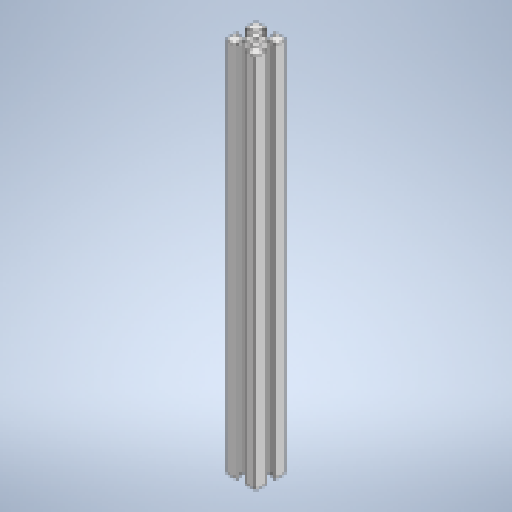
# Autodesk Inventor part: j2j3 alumi ext
Saved by Autodesk Inventor 2025 (Build 290162000, 162)
## iProperties
Created: 2025-07-28
Part Number: j2j3 alumi ext
Material: 一般
Document SubType Name: Modeling
Designer: gavin
Density: 1 g/cm^3
Appearance: 預設
Author: gavin
Autodesk Inventor part; units mm, degrees
ref_plane "YZ Plane" through (0, 0, 0) normal (1, 0, 0) x (0, 1, 0)
ref_plane "XZ Plane" through (0, 0, 0) normal (0, 1, 0) x (-1, 0, 0)
ref_plane "XY Plane" through (0, 0, 0) normal (0, 0, 1) x (1, 0, 0)
sketch "草圖1" plane through (0, 0, 0) normal (0, 1, 0) x (-1, 0, 0)
  line L0 (10, 10) -> (10, -10)
  line L1 (-10, -10) -> (-10, 10)
  line L2 (-10, 10) -> (10, -10) construction
  line L3 (10, 10) -> (-10, -10) construction
  line L4 (2.65, -10) -> (2.65, -8.5)
  line L5 (2.65, -8.5) -> (4.15, -8.5)
  line L6 (4.15, -8.5) -> (4.15, -4.9973)
  arc A0 (4.15, -4.9973) -> (-4.15, -4.9973) centre (0, -10) ccw
  line L7 (0, -10) -> (0, 0) construction
  line L8 (-2.65, -10) -> (-2.65, -8.5)
  line L9 (-2.65, -8.5) -> (-4.15, -8.5)
  line L10 (-4.15, -8.5) -> (-4.15, -4.9973)
  arc A1 (4.9973, 4.15) -> (4.9973, -4.15) centre (10, 0) ccw
  line L11 (10, 2.65) -> (8.5, 2.65)
  line L12 (8.5, 2.65) -> (8.5, 4.15)
  line L13 (8.5, 4.15) -> (4.9973, 4.15)
  line L14 (10, -2.65) -> (8.5, -2.65)
  line L15 (8.5, -2.65) -> (8.5, -4.15)
  line L16 (8.5, -4.15) -> (4.9973, -4.15)
  arc A2 (-4.15, 4.9973) -> (4.15, 4.9973) centre (0, 10) ccw
  line L17 (-2.65, 10) -> (-2.65, 8.5)
  line L18 (-2.65, 8.5) -> (-4.15, 8.5)
  line L19 (-4.15, 8.5) -> (-4.15, 4.9973)
  line L20 (2.65, 10) -> (2.65, 8.5)
  line L21 (2.65, 8.5) -> (4.15, 8.5)
  line L22 (4.15, 8.5) -> (4.15, 4.9973)
  arc A3 (-4.9973, -4.15) -> (-4.9973, 4.15) centre (-10, 0) ccw
  line L23 (-10, -2.65) -> (-8.5, -2.65)
  line L24 (-8.5, -2.65) -> (-8.5, -4.15)
  line L25 (-8.5, -4.15) -> (-4.9973, -4.15)
  line L26 (-10, 2.65) -> (-8.5, 2.65)
  line L27 (-8.5, 2.65) -> (-8.5, 4.15)
  line L28 (-8.5, 4.15) -> (-4.9973, 4.15)
  line L29 (10, -10) -> (2.65, -10)
  line L30 (-2.65, -10) -> (-10, -10)
  line L31 (-10, 10) -> (-2.65, 10)
  line L32 (2.65, 10) -> (10, 10)
  circle A4 centre (0, 0) radius 1.65
  point P0 (2.65, -9.25)
  point P1 (-2.65, -9.25)
  point P2 (9.25, 2.65)
  point P3 (9.25, -2.65)
  point P4 (-2.65, 9.25)
  point P5 (2.65, 9.25)
  point P6 (-9.25, -2.65)
  point P7 (-9.25, 2.65)
  dimension "d0" = 20
  dimension "d1" = 20
  dimension "d2" = 13
  dimension "d3" = 1.5
  dimension "d4" = 2.65
  dimension "d5" = 4.15
  dimension "d8" = 360
  dimension "d10" = 3.3
  constraints: 66 end point, 8 point on circle, 6 perpendicular, 5 centre point, 5 parallel, 5 symmetric about line, 3 midpoint, 2 horizontal, 1 coincident, 1 vertical, 73 other
  measures "d0" distance of L0.end L1.start
  measures "d1" distance of L0.start L0.end
  measures "d2" diameter of A0
  measures "d3" distance of L4.start L4.end
  measures "d4" distance from line of point (2.65, -9.25) L7
  measures "d5" distance between parallel lines of L7 L6
  measures "d10" diameter of A4
extrude "擠出1" add sketch "草圖1" along normal blind 250 contours L0 L11 L12 L13 A1 L16 L15 L14 L29 L4 L5 L6 A0 L10 L9 L8 L30 L1 L23 L24 L25 A3 L28 L27 L26 L31 L17 L18 L19 A2 L22 L21 L20 L32
